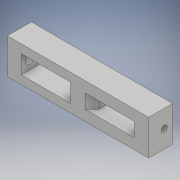
# Autodesk Inventor part: cage2table-mount-M4(top)-M6(bottom)-H100mm-HoleOffset5mm
Saved by Autodesk Inventor 2017 (Build 210142000, 142)
## iProperties
Created: 2022-06-20
Part Number: cage2table-mount-M4(top)-M6(bottom)-H100mm-HoleOffset5mm
Material: Generic
Document SubType Name: Modeling
Designer: Nikita
Density: 1 g/cm^3
Appearance: Default
Author: Nikita
Autodesk Inventor part; units mm, degrees
ref_plane "YZ Plane" through (0, 0, 0) normal (1, 0, 0) x (0, 1, 0)
ref_plane "XZ Plane" through (0, 0, 0) normal (0, 1, 0) x (-1, 0, 0)
ref_plane "XY Plane" through (0, 0, 0) normal (0, 0, 1) x (1, 0, 0)
sketch "Sketch1" plane through (0, 0, 0) normal (0, 0, 1) x (1, 0, 0)
  line L0 (50, -12.5) -> (-50, -12.5)
  line L1 (-50, -12.5) -> (-50, 12.5)
  line L2 (-50, 12.5) -> (50, 12.5)
  line L3 (50, 12.5) -> (50, -12.5)
  line L4 (50, -12.5) -> (-50, 12.5) construction
  line L5 (-50, -12.5) -> (50, 12.5) construction
  line L6 (-10, -5) -> (-40, -5)
  line L7 (-40, -5) -> (-40, 5)
  line L8 (-40, 5) -> (-10, 5)
  line L9 (-10, 5) -> (-10, -5)
  line L10 (-10, -5) -> (-40, 5) construction
  line L11 (-40, -5) -> (-10, 5) construction
  line L12 (10.2094, -6.5) -> (40.2094, -6.5)
  line L13 (40.2094, -6.5) -> (40.2094, 6.5)
  line L14 (40.2094, 6.5) -> (10.2094, 6.5)
  line L15 (10.2094, 6.5) -> (10.2094, -6.5)
  line L16 (10.2094, -6.5) -> (40.2094, 6.5) construction
  line L17 (40.2094, -6.5) -> (10.2094, 6.5) construction
  point P0 (0, 0)
  point P1 (-40, 0)
  point P2 (40, 0)
  point P3 (-25, 0)
  point P4 (25.2094, 0)
  dimension "d0" = 100
  dimension "d1" = 25
  dimension "d2" = 10
  dimension "d3" = 13
  constraints: 36 end point, 6 midpoint, 6 parallel, 4 perpendicular, 2 horizontal
  measures "d0" distance of L1.end L2.end
  measures "d1" distance of L0.end L1.end
  measures "d2" distance of L6.end L7.end
  measures "d3" distance of L13.end L12.end
extrude "Extrusion1" add sketch "Sketch1" along normal blind 17
sketch "M6 thru" plane through (50, -12.5, 0) normal (1, 0, 0) x (0, 0, -1)
  line L0 (0, 25) -> (0, 0) projected
  point P0 (0, 12.5)
  point P1 (-6, 12.5)
  dimension "d13" = 6
  measures "d13" distance from line of point (-6, 12.5) L0
sketch "Sketch3" plane through (-50, -12.5, 0) normal (-1, 0, 0) x (0, 0, 1)
  line L0 (0, 0) -> (0, 25) projected
  point P0 (0, 12.5)
  point P1 (11, 12.5)
  dimension "d14" = 11
  measures "d14" distance from line of L0 point (11, 12.5)
hole "M6 thru-hole" at (50, 0, 6) direction (-1, 0, 0) diameter 6.4 end up to face face through (40.2094, -2.1667, 11.3333) facing (-1, 0, 0)
hole "M4 thru-hole" at (-50, 0, 11) direction (1, 0, 0) diameter 4.4 end up to face face through (-40, 1.6667, 5.6667) facing (1, 0, 0)
chamfer "Chamfer1" distance 5 angle 45 4 edges at (-10, 0, 17) (10.2094, 0, 17) (-10, 0, 0) (10.2094, 0, 0)
body "Solid1"
